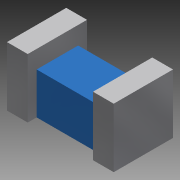
# Autodesk Inventor part: 0603Inductor
Saved by Autodesk Inventor 2014 (Build 180170000, 170)
## iProperties
Created: 2015-11-06
Part Number: 0603Inductor
Material: Generic
Document SubType Name: Modeling
Designer: Owner
Density: 1 g/cm^3
Appearance: Default
Author: Owner
Autodesk Inventor part; units mm, degrees
ref_plane "YZ Plane" through (0, 0, 0) normal (1, 0, 0) x (0, 1, 0)
ref_plane "XZ Plane" through (0, 0, 0) normal (0, 1, 0) x (-1, 0, 0)
ref_plane "XY Plane" through (0, 0, 0) normal (0, 0, 1) x (1, 0, 0)
sketch "Sketch1" plane through (0, 0, 0) normal (0, 1, 0) x (-1, 0, 0)
  line L0 (-0.7794, 0.3056) -> (0.8206, 0.3056)
  line L1 (0.8206, 0.3056) -> (0.8206, -0.3944)
  line L2 (0.8206, -0.3944) -> (-0.7794, -0.3944)
  line L3 (-0.7794, -0.3944) -> (-0.7794, 0.3056)
  point P0 (0, 0)
  dimension "d0" = 1.6
  dimension "d1" = 0.7
  constraints: 8 end point, 2 parallel, 1 horizontal, 1 perpendicular
  measures "d0" distance of L0.start L0.end
  measures "d1" distance of L0.end L1.end
extrude "Extrusion1" add sketch "Sketch1" along normal blind 0.7
sketch "Sketch2" plane through (0, 0, 0) normal (0, -1, 0) x (1, 0, 0)
  line L0 (0.7794, 0.3056) -> (-0.8206, 0.3056) projected
  line L1 (-0.8206, 0.3056) -> (-0.8206, -0.3944) projected
  line L2 (-0.9206, 0.4556) -> (-0.5706, 0.4556)
  line L3 (-0.5706, 0.4556) -> (-0.5706, -0.5444)
  line L4 (-0.5706, -0.5444) -> (-0.9206, -0.5444)
  line L5 (-0.9206, -0.5444) -> (-0.9206, 0.4556)
  line L6 (0.5294, 0.4556) -> (0.8794, 0.4556)
  line L7 (0.8794, 0.4556) -> (0.8794, -0.5444)
  line L8 (0.8794, -0.5444) -> (0.5294, -0.5444)
  line L9 (0.5294, -0.5444) -> (0.5294, 0.4556)
  point P0 (0, 0)
  dimension "d4" = 0.35
  dimension "d5" = 0.35
  dimension "d6" = 1.8
  dimension "d7" = 0.1
  dimension "d8" = 1
  dimension "d9" = 1
  dimension "d10" = 0.15
  dimension "d11" = 0.15
  constraints: 16 end point, 4 parallel, 2 horizontal, 2 perpendicular
  measures "d4" distance of L2.start L2.end
  measures "d5" distance of L6.start L6.end
  measures "d6" distance between parallel lines of L7 L5
  measures "d7" distance between parallel lines of L1 L5
  measures "d8" distance of L4.end L2.start
  measures "d9" distance of L6.end L7.end
  measures "d10" distance between parallel lines of L0 L6
  measures "d11" distance between parallel lines of L0 L2
extrude "Extrusion2" add sketch "Sketch2" against normal blind 1
body "Solid1"
